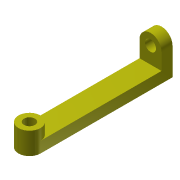
# Autodesk Inventor part: 本體
Saved by Autodesk Inventor 2015 SP2 (Build 190223200, 223)
## iProperties
Created: 2020-03-26
Part Number: 本體
Material: 一般
Document SubType Name: Modeling
Designer: Kuan-Lun Hsu
Density: 1 g/cm^3
Appearance: 黃
Author: Kuan-Lun Hsu
Autodesk Inventor part; units mm, degrees
ref_plane "YZ Plane" through (0, 0, 0) normal (1, 0, 0) x (0, 1, 0)
ref_plane "XZ Plane" through (0, 0, 0) normal (0, 1, 0) x (-1, 0, 0)
ref_plane "XY Plane" through (0, 0, 0) normal (0, 0, 1) x (1, 0, 0)
sketch "草圖1" plane through (0, 0, 0) normal (0, 0, 1) x (1, 0, 0)
  line L0 (-10, 120) -> (10, 120)
  line L1 (10, 120) -> (10, -20)
  line L2 (10, -20) -> (-10, -20)
  line L3 (-10, -20) -> (-10, 120)
  point P0 (0, 0)
  point P1 (0, -20)
  dimension "d0" = 20
  dimension "d1" = 140
  dimension "d2" = 20
  constraints: 8 end point, 2 parallel, 1 horizontal, 1 midpoint, 1 perpendicular, 1 vertical alignment
  measures "d0" distance from line of L2 point (0, 0)
  measures "d1" distance of L2.end L0.start
  measures "d2" distance of L0.start L0.end
extrude "擠出1" add sketch "草圖1" along normal blind 10
sketch "草圖2" plane through (0, 0, 10) normal (0, 0, 1) x (1, 0, 0)
  circle A0 centre (0, 0) radius 10
  circle A1 centre (0, 0) radius 5
  dimension "d5" = 20
  dimension "d6" = 10
  constraints: 2 centre point, 2 coincident
  measures "d5" diameter of A0
  measures "d6" diameter of A1
extrude "擠出2" add sketch "草圖2" along normal blind 10
sketch "草圖3" plane through (-10, 120, 0) normal (0, 1, 0) x (1, 0, 0)
  circle A0 centre (10, -25) radius 10
  line L0 (20, -10) -> (0, -10) projected
  line L1 (0, 0) -> (20, 0) projected
  line L2 (0, 0) -> (20, 0)
  line L3 (20, 0) -> (20, -25)
  line L4 (20, -25) -> (0, -25)
  line L5 (0, -25) -> (0, 0)
  point P0 (10, 0)
  point P1 (10, -10)
  point P2 (10, 0)
  dimension "d9" = 20
  dimension "d10" = 25
  constraints: 8 end point, 3 midpoint, 2 parallel, 1 horizontal, 1 horizontal alignment, 1 perpendicular, 1 vertical, 1 vertical alignment, 2 other
  measures "d10" distance from line of L1 point (10, -25)
extrude "擠出3" add sketch "草圖3" against normal blind 10
sketch "草圖4" plane through (-10, 120, 0) normal (0, 1, 0) x (1, 0, 0)
  arc A0 (0, -25) -> (20, -25) centre (10, -25) ccw projected
  circle A1 centre (10, -25) radius 5
  point P0 (10, 0)
  dimension "d13" = 10
  constraints: 1 centre point, 1 coincident
  measures "d13" diameter of A1
extrude "擠出4" cut sketch "草圖4" against normal blind 10
sketch "草圖5" plane through (0, 0, 10) normal (0, 0, 1) x (1, 0, 0)
  arc A0 (-10, 0) -> (10, 0) centre (0, 0) ccw projected
  line L0 (-10, 0) -> (-10, -20) projected
  line L1 (-10, -20) -> (10, -20) projected
  line L2 (10, -20) -> (10, 0) projected
extrude "擠出5" cut sketch "草圖5" against normal through all
